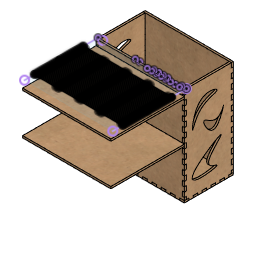
laser_skurdur_hlutur (Autodesk Fusion 360 design; units mm, degrees)
Autodesk Fusion 360 part; units mm, degrees
note: some values were not read from the file. Set by a fixed rule: which sketch regions a step uses.
sketch "botn sketch" plane through (0, 0, 0) normal (0, 0, 1) x (1, 0, 0)
  line L0 (0, 0) -> (180, 0)
  line L1 (180, 0) -> (180, 100)
  line L2 (180, 100) -> (0, 100)
  line L3 (0, 100) -> (0, 0)
  dimension "d16" = 180
  dimension "d17" = 100
  constraint horizontal L0
  constraint vertical L1
  constraint horizontal L2
  constraint vertical L3
  constraint coincident L0.start L3.end
  measures "d16" distance of L0.start L0.end
  measures "d17" distance of L0.start L2.end
extrude "Extrude1" add sketch "botn sketch" along normal blind 4 makes body 1
sketch "botn front fingur sketch" plane through (0, 0, 0) normal (0, -1, 0) x (1, 0, 0)
  line L0 (0, 0) -> (180, 0)
  line L1 (180, 0) -> (180, 4)
  line L2 (180, 4) -> (0, 4)
  line L3 (0, 4) -> (0, 0)
  line L4 (9.4737, 0) -> (18.9474, 0)
  line L5 (18.9474, 0) -> (18.9474, 4)
  line L6 (18.9474, 4) -> (9.4737, 4)
  line L7 (9.4737, 4) -> (9.4737, 0)
  dimension "d20" = 9.4737
  dimension "d21" = 9.4737
  constraint horizontal L4
  constraint vertical L5
  constraint horizontal L6
  constraint vertical L7
  constraint coincident L2 L5.end
  constraint coincident L0 L4.start
  measures "d20" distance of L5.end L6.end
  measures "d21" distance of L3 L7
extrude "Extrude2" cut sketch "botn front fingur sketch" against normal blind 4 contours L0 L2 L4 L5 L6 L7 bodies 1
pattern_linear "R-Pattern1" count 9 spacing 18.9474 along (1, 0, 0) of "Extrude2"
sketch "afturhlid sketch" plane through (0, 0, 0) normal (0, 1, 0) x (1, 0, 0)
  line L0 (0, 0) -> (180, 0)
  line L1 (180, 0) -> (180, -200)
  line L2 (180, -200) -> (0, -200)
  line L3 (0, -200) -> (0, 0)
  point P0 (180, 0)
  dimension "d28" = 200
  constraint perpendicular L0 L1
  constraint parallel L0 L2
  constraint parallel L1 L3
  constraint coincident P0 L0.end
  constraint horizontal L0
  constraint coincident L0.start L3.end
  measures "d28" distance of L0.start L2.end
extrude "Extrude3" add sketch "afturhlid sketch" along normal blind 4 separate body makes body 2
combine "Combine1" operation cut target body 2 tool bodies 1 keep tools
sketch "afturhlid vinstri sketch" plane through (0, 0, 0) normal (-1, 0, 0) x (0, -1, 0)
  line L0 (-4, 4) -> (0, 4)
  line L1 (0, 4) -> (0, 200)
  line L2 (0, 200) -> (-4, 200)
  line L3 (-4, 200) -> (-4, 4)
  line L4 (0, 9.5238) -> (-4, 9.5238)
  line L5 (-4, 9.5238) -> (-4, 19.0476)
  line L6 (-4, 19.0476) -> (0, 19.0476)
  line L7 (0, 19.0476) -> (0, 9.5238)
  dimension "d31" = 9.5238
  dimension "d32" = 9.5238
  constraint horizontal L4
  constraint vertical L5
  constraint horizontal L6
  constraint vertical L7
  constraint coincident L3 L5.end
  constraint coincident L1 L4.start
  measures "d31" distance of L4.start L6.end
  measures "d32" distance of origin L4
extrude "Extrude4" cut sketch "afturhlid vinstri sketch" against normal blind 4 contours L1 L3 L4 L5 L6 L7 bodies 2
pattern_linear "R-Pattern2" count 10 spacing 19.0476 along (0, 0, 1) of "Extrude4"
extrude "Extrude5" add 1 faces at (99.2281, 4, 106.0952) along direction (0, -1, 0) blind 4 from surface at -96 separate body on bodies 2 makes body 3
combine "Combine2" operation cut target body 1 tool bodies 3 keep tools
sketch "hlid sketch" plane through (0, 0, 0) normal (1, 0, 0) x (0, 1, 0)
  line L0 (0, 0) -> (100, 0)
  line L1 (100, 0) -> (100, 200)
  line L2 (100, 200) -> (0, 200)
  line L3 (0, 200) -> (0, 0)
  dimension "d42" = 100
  dimension "d43" = 200
  constraint horizontal L0
  constraint vertical L1
  constraint horizontal L2
  constraint vertical L3
  constraint coincident L0.start L3.end
  measures "d42" distance of L0.start L0.end
  measures "d43" distance of L0.start L2.end
extrude "Extrude6" add sketch "hlid sketch" along normal blind 4 separate body makes body 4
sketch "hlid_botn fingur sketch" plane through (0, 0, 0) normal (-1, 0, 0) x (0, -1, 0)
  line L0 (-100, 0) -> (0, 0)
  line L1 (0, 0) -> (0, 4)
  line L2 (0, 4) -> (-100, 4)
  line L3 (-100, 4) -> (-100, 0)
  line L4 (-9.0909, 0) -> (-18.1818, 0)
  line L5 (-18.1818, 0) -> (-18.1818, 4)
  line L6 (-18.1818, 4) -> (-9.0909, 4)
  line L7 (-9.0909, 4) -> (-9.0909, 0)
  dimension "d46" = 9.0909
  dimension "d47" = 9.0909
  constraint horizontal L4
  constraint vertical L5
  constraint horizontal L6
  constraint vertical L7
  constraint coincident L2 L5.end
  constraint coincident L0 L4.start
  measures "d46" distance of L4.start L4.end
  measures "d47" distance of L0.end L7
extrude "Extrude7" cut sketch "hlid_botn fingur sketch" against normal blind 4 contours L0 L2 L4 L5 L6 L7 bodies 1
pattern_linear "R-Pattern3" count 5 spacing 18.1818 along (0, 1, 0) of "Extrude7"
combine "Combine3" operation cut target body 4 tool bodies 3 2 1 keep tools
extrude "Extrude8" add 1 faces at (4, 51.5152, 33.0794) along direction (-1, 0, 0) blind 4 from surface at -176 separate body on bodies 4 makes body 5
combine "Combine4" operation cut target body 2 tool bodies 5 keep tools
combine "Combine5" operation cut target body 1 tool bodies 5 keep tools
combine "Combine6" operation cut target body 3 tool bodies 5 keep tools
sketch "living hinge fyrsta sketch" plane through (0, 4, 0) normal (0, 1, 0) x (-1, 0, 0)
  line L0 (-176, 190.4762) -> (-176, 180.9524)
  line L1 (-176, 47.619) -> (-180, 47.619)
  line L2 (-180, 180.9524) -> (-180, 171.4286)
  line L3 (-180, 38.0952) -> (-176, 38.0952)
  line L4 (-176, 38.0952) -> (-176, 28.5714)
  line L5 (-176, 28.5714) -> (-180, 28.5714)
  line L6 (-180, 28.5714) -> (-180, 19.0476)
  line L7 (-180, 19.0476) -> (-176, 19.0476)
  line L8 (-176, 19.0476) -> (-176, 9.5238)
  line L9 (-176, 9.5238) -> (-180, 9.5238)
  line L10 (-180, 9.5238) -> (-180, 4)
  line L11 (-180, 4) -> (-170.5263, 4)
  line L12 (-94.7368, 4) -> (-94.7368, 0)
  line L13 (-170.5263, 0) -> (-161.0526, 0)
  line L14 (-85.2632, 0) -> (-85.2632, 4)
  line L15 (-85.2632, 4) -> (-75.7895, 4)
  line L16 (-75.7895, 4) -> (-75.7895, 0)
  line L17 (-75.7895, 0) -> (-66.3158, 0)
  line L18 (-66.3158, 0) -> (-66.3158, 4)
  line L19 (-66.3158, 4) -> (-56.8421, 4)
  line L20 (-56.8421, 4) -> (-56.8421, 0)
  line L21 (-56.8421, 0) -> (-47.3684, 0)
  line L22 (-47.3684, 0) -> (-47.3684, 4)
  line L23 (-47.3684, 4) -> (-37.8947, 4)
  line L24 (-37.8947, 4) -> (-37.8947, 0)
  line L25 (-37.8947, 0) -> (-28.4211, 0)
  line L26 (-28.4211, 0) -> (-28.4211, 4)
  line L27 (-28.4211, 4) -> (-18.9474, 4)
  line L28 (-18.9474, 4) -> (-18.9474, 0)
  line L29 (-18.9474, 0) -> (-9.4737, 0)
  line L30 (-9.4737, 0) -> (-9.4737, 4)
  line L31 (-9.4737, 4) -> (0, 4)
  line L32 (0, 4) -> (0, 9.5238)
  line L33 (0, 9.5238) -> (-4, 9.5238)
  line L34 (-4, 9.5238) -> (-4, 19.0476)
  line L35 (-4, 19.0476) -> (0, 19.0476)
  line L36 (0, 19.0476) -> (0, 28.5714)
  line L37 (0, 28.5714) -> (-4, 28.5714)
  line L38 (-4, 28.5714) -> (-4, 38.0952)
  line L39 (-4, 38.0952) -> (0, 38.0952)
  line L40 (0, 38.0952) -> (0, 47.619)
  line L41 (0, 47.619) -> (-4, 47.619)
  line L42 (-4, 47.619) -> (-4, 57.1429)
  line L43 (-4, 57.1429) -> (0, 57.1429)
  line L44 (0, 57.1429) -> (0, 66.6667)
  line L45 (0, 200) -> (-180, 200)
  line L46 (-180, 200) -> (-180, 190.4762)
  line L47 (-180, 57.1429) -> (-176, 57.1429)
  line L48 (0, 200) -> (-180, 200)
  line L49 (-180, 200) -> (-180, 196)
  line L50 (-180, 196) -> (0, 196)
  line L51 (0, 196) -> (0, 200)
  line L52 (-176, 85.7143) -> (-180, 85.7143)
  line L53 (-180, 76.1905) -> (-176, 76.1905)
  line L54 (-176, 76.1905) -> (-176, 66.6667)
  line L55 (-176, 66.6667) -> (-180, 66.6667)
  line L56 (-180, 66.6667) -> (-180, 57.1429)
  line L57 (0, 66.6667) -> (-4, 66.6667)
  line L58 (-4, 66.6667) -> (-4, 76.1905)
  line L59 (-4, 76.1905) -> (0, 76.1905)
  line L60 (0, 76.1905) -> (0, 85.7143)
  line L61 (0, 85.7143) -> (-4, 85.7143)
  line L62 (-4, 85.7143) -> (-4, 95.2381)
  line L63 (-4, 95.2381) -> (0, 95.2381)
  line L64 (0, 95.2381) -> (0, 104.7619)
  line L65 (-180, 95.2381) -> (-176, 95.2381)
  line L66 (-176, 180.9524) -> (-180, 180.9524)
  line L67 (-180, 171.4286) -> (-176, 171.4286)
  line L68 (-176, 171.4286) -> (-176, 161.9048)
  line L69 (-176, 161.9048) -> (-180, 161.9048)
  line L70 (-180, 161.9048) -> (-180, 152.381)
  line L71 (-180, 152.381) -> (-176, 152.381)
  line L72 (-176, 152.381) -> (-176, 142.8571)
  line L73 (-176, 142.8571) -> (-180, 142.8571)
  line L74 (-180, 142.8571) -> (-180, 133.3333)
  line L75 (-180, 133.3333) -> (-176, 133.3333)
  line L76 (-176, 133.3333) -> (-176, 123.8095)
  line L77 (-176, 123.8095) -> (-180, 123.8095)
  line L78 (-180, 123.8095) -> (-180, 114.2857)
  line L79 (-180, 114.2857) -> (-176, 114.2857)
  line L80 (-176, 114.2857) -> (-176, 104.7619)
  line L81 (-176, 104.7619) -> (-180, 104.7619)
  line L82 (-180, 104.7619) -> (-180, 95.2381)
  line L83 (-176, 95.2381) -> (-176, 85.7143)
  line L84 (-180, 85.7143) -> (-180, 76.1905)
  line L85 (0, 104.7619) -> (-4, 104.7619)
  line L86 (-4, 104.7619) -> (-4, 114.2857)
  line L87 (-4, 114.2857) -> (0, 114.2857)
  line L88 (0, 114.2857) -> (0, 123.8095)
  line L89 (0, 123.8095) -> (-4, 123.8095)
  line L90 (-4, 123.8095) -> (-4, 133.3333)
  line L91 (-4, 133.3333) -> (0, 133.3333)
  line L92 (0, 133.3333) -> (0, 142.8571)
  line L93 (0, 142.8571) -> (-4, 142.8571)
  line L94 (-4, 142.8571) -> (-4, 152.381)
  line L95 (-4, 152.381) -> (0, 152.381)
  line L96 (0, 152.381) -> (0, 161.9048)
  line L97 (0, 161.9048) -> (-4, 161.9048)
  line L98 (-4, 161.9048) -> (-4, 171.4286)
  line L99 (-4, 171.4286) -> (0, 171.4286)
  line L100 (0, 171.4286) -> (0, 180.9524)
  line L101 (0, 180.9524) -> (-4, 180.9524)
  line L102 (-4, 180.9524) -> (-4, 190.4762)
  line L103 (-4, 190.4762) -> (0, 190.4762)
  line L104 (0, 190.4762) -> (0, 200)
  line L105 (-180, 190.4762) -> (-176, 190.4762)
  line L106 (-176, 57.1429) -> (-176, 47.619)
  line L107 (-180, 47.619) -> (-180, 38.0952)
  line L108 (-170.5263, 4) -> (-170.5263, 0)
  line L109 (-161.0526, 0) -> (-161.0526, 4)
  line L110 (-161.0526, 4) -> (-151.5789, 4)
  line L111 (-151.5789, 4) -> (-151.5789, 0)
  line L112 (-151.5789, 0) -> (-142.1053, 0)
  line L113 (-142.1053, 0) -> (-142.1053, 4)
  line L114 (-142.1053, 4) -> (-132.6316, 4)
  line L115 (-132.6316, 4) -> (-132.6316, 0)
  line L116 (-132.6316, 0) -> (-123.1579, 0)
  line L117 (-123.1579, 0) -> (-123.1579, 4)
  line L118 (-123.1579, 4) -> (-113.6842, 4)
  line L119 (-113.6842, 4) -> (-113.6842, 0)
  line L120 (-113.6842, 0) -> (-104.2105, 0)
  line L121 (-104.2105, 0) -> (-104.2105, 4)
  line L122 (-104.2105, 4) -> (-94.7368, 4)
  line L123 (-94.7368, 0) -> (-85.2632, 0)
  point P0 (0, 200)
  dimension "d57" = 180
  dimension "d58" = 4
  constraint horizontal L48
  constraint vertical L49
  constraint horizontal L50
  constraint vertical L51
  constraint coincident P0 L45.start
  measures "d57" distance of P0 L45.end
  measures "d58" distance of P0 L50.end
extrude "Extrude9" add sketch "living hinge fyrsta sketch" against normal blind 150 separate body contours L45 L46 L48 L49 L50 L51 L104 makes body 6
sketch "living hinge annad sketch" plane through (0, 4, 0) normal (0, 1, 0) x (-1, 0, 0)
  line L0 (0, 196) -> (0, 200)
  line L1 (0, 200) -> (-180, 200)
  line L2 (-180, 200) -> (-180, 196)
  line L3 (-180, 196) -> (0, 196)
  line L4 (-9.4737, 200) -> (-18.9474, 200)
  line L5 (-18.9474, 200) -> (-18.9474, 196)
  line L6 (-18.9474, 196) -> (-9.4737, 196)
  line L7 (-9.4737, 196) -> (-9.4737, 200)
  dimension "d62" = 9.4737
  dimension "d63" = 9.4737
  constraint horizontal L4
  constraint vertical L5
  constraint horizontal L6
  constraint vertical L7
  constraint coincident L3 L5.end
  constraint coincident L1 L4.start
  measures "d62" distance of L4.start L4.end
  measures "d63" distance of origin L7
extrude "Extrude10" cut sketch "living hinge annad sketch" against normal blind 4 contours L1 L3 L4 L5 L6 L7 bodies 6
pattern_linear "R-Pattern4" count 9 spacing 18.9474 along (1, 0, 0) of "Extrude10"
sketch "living hinge adal sketch" plane through (0, 0, 200) normal (0, 0, 1) x (-1, 0, 0)
  line L0 (-85.2632, 0) -> (-85.2632, -4)
  line L1 (-161.0526, -4) -> (-151.5789, -4)
  line L2 (-75.7895, -4) -> (-75.7895, 0)
  line L3 (-75.7895, 0) -> (-66.3158, 0)
  line L4 (-66.3158, 0) -> (-66.3158, -4)
  line L5 (-66.3158, -4) -> (-56.8421, -4)
  line L6 (-56.8421, -4) -> (-56.8421, 0)
  line L7 (-56.8421, 0) -> (-47.3684, 0)
  line L8 (-47.3684, 0) -> (-47.3684, -4)
  line L9 (-47.3684, -4) -> (-37.8947, -4)
  line L10 (-37.8947, -4) -> (-37.8947, 0)
  line L11 (-37.8947, 0) -> (-28.4211, 0)
  line L12 (-28.4211, 0) -> (-28.4211, -4)
  line L13 (-28.4211, -4) -> (-18.9474, -4)
  line L14 (-18.9474, -4) -> (-18.9474, 0)
  line L15 (-18.9474, 0) -> (-9.4737, 0)
  line L16 (-9.4737, 0) -> (-9.4737, -4)
  line L17 (-9.4737, -4) -> (0, -4)
  line L18 (0, -4) -> (0, 146) construction
  line L19 (0, 146) -> (-180, 146)
  line L20 (-180, 146) -> (-180, -4)
  line L21 (-104.2105, -4) -> (-94.7368, -4)
  line L22 (-94.7368, -4) -> (-94.7368, 0)
  line L23 (-94.7368, 0) -> (-85.2632, 0)
  line L24 (0, 26) -> (-180, 26) construction
  line L25 (0, 126) -> (-180, 126) construction
  line L26 (0, 76) -> (-180, 76) construction
  line L27 (0, -4) -> (-9.4737, -4) construction
  line L28 (-180, -4) -> (-180, 146)
  line L29 (0, -4) -> (0, 146)
  line L30 (0.5, 26) -> (-43.5, 26)
  line L31 (-49.5, 26) -> (-130.5, 26)
  line L32 (-6, 28) -> (-87, 28)
  line L33 (-93, 28) -> (-174, 28)
  line L34 (-136.5, 26) -> (-180.5, 26)
  line L35 (-90, 76) -> (-90, 26) construction
  line L36 (-46.5, 28) -> (-43.5, 26) construction
  line L37 (-46.5, 28) -> (-49.5, 26) construction
  line L38 (0.5, 126) -> (-43.5, 126)
  line L39 (-49.5, 126) -> (-130.5, 126)
  line L40 (-136.5, 126) -> (-180.5, 126)
  line L41 (0.5, 30) -> (-43.5, 30)
  line L42 (-6, 32) -> (-87, 32)
  line L43 (-49.5, 30) -> (-130.5, 30)
  line L44 (-93, 32) -> (-174, 32)
  line L45 (-136.5, 30) -> (-180.5, 30)
  line L46 (0.5, 34) -> (-43.5, 34)
  line L47 (-6, 36) -> (-87, 36)
  line L48 (-49.5, 34) -> (-130.5, 34)
  line L49 (-93, 36) -> (-174, 36)
  line L50 (-136.5, 34) -> (-180.5, 34)
  line L51 (0.5, 38) -> (-43.5, 38)
  line L52 (-6, 40) -> (-87, 40)
  line L53 (-49.5, 38) -> (-130.5, 38)
  line L54 (-93, 40) -> (-174, 40)
  line L55 (-136.5, 38) -> (-180.5, 38)
  line L56 (0.5, 42) -> (-43.5, 42)
  line L57 (-6, 44) -> (-87, 44)
  line L58 (-49.5, 42) -> (-130.5, 42)
  line L59 (-93, 44) -> (-174, 44)
  line L60 (-136.5, 42) -> (-180.5, 42)
  line L61 (0.5, 46) -> (-43.5, 46)
  line L62 (-6, 48) -> (-87, 48)
  line L63 (-49.5, 46) -> (-130.5, 46)
  line L64 (-93, 48) -> (-174, 48)
  line L65 (-136.5, 46) -> (-180.5, 46)
  line L66 (0.5, 50) -> (-43.5, 50)
  line L67 (-6, 52) -> (-87, 52)
  line L68 (-49.5, 50) -> (-130.5, 50)
  line L69 (-93, 52) -> (-174, 52)
  line L70 (-136.5, 50) -> (-180.5, 50)
  line L71 (0.5, 54) -> (-43.5, 54)
  line L72 (-6, 56) -> (-87, 56)
  line L73 (-49.5, 54) -> (-130.5, 54)
  line L74 (-93, 56) -> (-174, 56)
  line L75 (-136.5, 54) -> (-180.5, 54)
  line L76 (0.5, 58) -> (-43.5, 58)
  line L77 (-6, 60) -> (-87, 60)
  line L78 (-49.5, 58) -> (-130.5, 58)
  line L79 (-93, 60) -> (-174, 60)
  line L80 (-136.5, 58) -> (-180.5, 58)
  line L81 (0.5, 62) -> (-43.5, 62)
  line L82 (-6, 64) -> (-87, 64)
  line L83 (-49.5, 62) -> (-130.5, 62)
  line L84 (-93, 64) -> (-174, 64)
  line L85 (-136.5, 62) -> (-180.5, 62)
  line L86 (0.5, 66) -> (-43.5, 66)
  line L87 (-6, 68) -> (-87, 68)
  line L88 (-49.5, 66) -> (-130.5, 66)
  line L89 (-93, 68) -> (-174, 68)
  line L90 (-136.5, 66) -> (-180.5, 66)
  line L91 (0.5, 70) -> (-43.5, 70)
  line L92 (-6, 72) -> (-87, 72)
  line L93 (-49.5, 70) -> (-130.5, 70)
  line L94 (-93, 72) -> (-174, 72)
  line L95 (-136.5, 70) -> (-180.5, 70)
  line L96 (0.5, 74) -> (-43.5, 74)
  line L97 (-6, 76) -> (-87, 76)
  line L98 (-49.5, 74) -> (-130.5, 74)
  line L99 (-93, 76) -> (-174, 76)
  line L100 (-136.5, 74) -> (-180.5, 74)
  line L101 (0.5, 78) -> (-43.5, 78)
  line L102 (-6, 80) -> (-87, 80)
  line L103 (-49.5, 78) -> (-130.5, 78)
  line L104 (-93, 80) -> (-174, 80)
  line L105 (-136.5, 78) -> (-180.5, 78)
  line L106 (0.5, 82) -> (-43.5, 82)
  line L107 (-6, 84) -> (-87, 84)
  line L108 (-49.5, 82) -> (-130.5, 82)
  line L109 (-93, 84) -> (-174, 84)
  line L110 (-136.5, 82) -> (-180.5, 82)
  line L111 (0.5, 86) -> (-43.5, 86)
  line L112 (-6, 88) -> (-87, 88)
  line L113 (-49.5, 86) -> (-130.5, 86)
  line L114 (-93, 88) -> (-174, 88)
  line L115 (-136.5, 86) -> (-180.5, 86)
  line L116 (0.5, 90) -> (-43.5, 90)
  line L117 (-6, 92) -> (-87, 92)
  line L118 (-49.5, 90) -> (-130.5, 90)
  line L119 (-93, 92) -> (-174, 92)
  line L120 (-136.5, 90) -> (-180.5, 90)
  line L121 (0.5, 94) -> (-43.5, 94)
  line L122 (-6, 96) -> (-87, 96)
  line L123 (-49.5, 94) -> (-130.5, 94)
  line L124 (-93, 96) -> (-174, 96)
  line L125 (-136.5, 94) -> (-180.5, 94)
  line L126 (0.5, 98) -> (-43.5, 98)
  line L127 (-6, 100) -> (-87, 100)
  line L128 (-49.5, 98) -> (-130.5, 98)
  line L129 (-93, 100) -> (-174, 100)
  line L130 (-136.5, 98) -> (-180.5, 98)
  line L131 (0.5, 102) -> (-43.5, 102)
  line L132 (-6, 104) -> (-87, 104)
  line L133 (-49.5, 102) -> (-130.5, 102)
  line L134 (-93, 104) -> (-174, 104)
  line L135 (-136.5, 102) -> (-180.5, 102)
  line L136 (0.5, 106) -> (-43.5, 106)
  line L137 (-6, 108) -> (-87, 108)
  line L138 (-49.5, 106) -> (-130.5, 106)
  line L139 (-93, 108) -> (-174, 108)
  line L140 (-136.5, 106) -> (-180.5, 106)
  line L141 (0.5, 110) -> (-43.5, 110)
  line L142 (-6, 112) -> (-87, 112)
  line L143 (-49.5, 110) -> (-130.5, 110)
  line L144 (-93, 112) -> (-174, 112)
  line L145 (-136.5, 110) -> (-180.5, 110)
  line L146 (0.5, 114) -> (-43.5, 114)
  line L147 (-6, 116) -> (-87, 116)
  line L148 (-49.5, 114) -> (-130.5, 114)
  line L149 (-93, 116) -> (-174, 116)
  line L150 (-136.5, 114) -> (-180.5, 114)
  line L151 (0.5, 118) -> (-43.5, 118)
  line L152 (-6, 120) -> (-87, 120)
  line L153 (-49.5, 118) -> (-130.5, 118)
  line L154 (-93, 120) -> (-174, 120)
  line L155 (-136.5, 118) -> (-180.5, 118)
  line L156 (0.5, 122) -> (-43.5, 122)
  line L157 (-6, 124) -> (-87, 124)
  line L158 (-49.5, 122) -> (-130.5, 122)
  line L159 (-93, 124) -> (-174, 124)
  line L160 (-136.5, 122) -> (-180.5, 122)
  line L161 (-161.0526, 0) -> (-161.0526, -4)
  line L162 (-151.5789, -4) -> (-151.5789, 0)
  line L163 (-151.5789, 0) -> (-142.1053, 0)
  line L164 (-142.1053, 0) -> (-142.1053, -4)
  line L165 (-142.1053, -4) -> (-132.6316, -4)
  line L166 (-132.6316, -4) -> (-132.6316, 0)
  line L167 (-132.6316, 0) -> (-123.1579, 0)
  line L168 (-123.1579, 0) -> (-123.1579, -4)
  line L169 (-123.1579, -4) -> (-113.6842, -4)
  line L170 (-113.6842, -4) -> (-113.6842, 0)
  line L171 (-113.6842, 0) -> (-104.2105, 0)
  line L172 (-104.2105, 0) -> (-104.2105, -4)
  line L173 (-85.2632, -4) -> (-75.7895, -4)
  line L174 (-180, -4) -> (-170.5263, -4)
  line L175 (-170.5263, -4) -> (-170.5263, 0)
  line L176 (-170.5263, 0) -> (-161.0526, 0)
  dimension "d72" = 30
  dimension "d73" = 100
  dimension "d76" = 6
  dimension "d77" = 6
  dimension "d78" = 6
  dimension "d79" = 0.5
  dimension "d80" = 0.5
  dimension "d81" = 6
  dimension "d82" = 6
  dimension "d85" = 2
  dimension "d88" = 0
  dimension "d89" = 4
  constraint parallel L24 L25
  constraint parallel L25 L26
  constraint vertical L24.start L26.start
  constraint vertical L25.start L26.start
  constraint parallel L24 L27
  constraint symmetric L24 L25 L26
  constraint vertical L24.end L26.end
  constraint vertical L25.end L26.end
  constraint coincident L20 L24.end
  constraint coincident L18 L26.start
  constraint collinear L24 L30
  constraint collinear L24 L31
  constraint collinear L24 L34
  constraint midpoint L26 L35.start
  constraint perpendicular L31 L35
  constraint midpoint L31 L35.end
  constraint coincident L24 L31.start
  constraint horizontal L32
  constraint collinear L32 L33
  constraint symmetric L32.end L33.start L35
  constraint coincident L24 L30.end
  constraint midpoint L32 L36.start
  constraint equal L36 L37
  constraint symmetric L26 L30.start L38.start
  constraint symmetric L26 L30.end L38.end
  constraint symmetric L26 L31.start L39.start
  constraint symmetric L26 L31.end L39.end
  constraint symmetric L26 L34.start L40.start
  constraint symmetric L26 L34.end L40.end
  measures "d72" distance of L24 L27
  measures "d73" distance of L24 L25
  measures "d76" distance of L30.end L31.start
  measures "d77" distance of L31.end L34.start
  measures "d78" distance of L32.end L33.start
  measures "d79" distance of L24.start L30.start
  measures "d80" distance of L20 L34.end
  measures "d81" horizontal distance of L24.start L32.start
  measures "d82" horizontal distance of L24.end L33.end
  measures "d85" distance of L30 L32
sketch "list2" plane through (0, 0, 0) normal (-1, 0, 0) x (0, -1, 0)
  line L0 (-96, 4) -> (-90.9091, 4)
  line L1 (-54.5455, 4) -> (-54.5455, 0)
  line L2 (-90.9091, 0) -> (-81.8182, 0)
  line L3 (-45.4545, 0) -> (-45.4545, 4)
  line L4 (-45.4545, 4) -> (-36.3636, 4)
  line L5 (-36.3636, 4) -> (-36.3636, 0)
  line L6 (-36.3636, 0) -> (-27.2727, 0)
  line L7 (-27.2727, 0) -> (-27.2727, 4)
  line L8 (-27.2727, 4) -> (-18.1818, 4)
  line L9 (-18.1818, 4) -> (-18.1818, 0)
  line L10 (-18.1818, 0) -> (-9.0909, 0)
  line L11 (-9.0909, 0) -> (-9.0909, 4)
  line L12 (-9.0909, 4) -> (-4, 4)
  line L13 (-4, 4) -> (-4, 9.5238)
  line L14 (-4, 9.5238) -> (0, 9.5238)
  line L15 (0, 9.5238) -> (0, 19.0476)
  line L16 (0, 19.0476) -> (-4, 19.0476)
  line L17 (-4, 19.0476) -> (-4, 28.5714)
  line L18 (-4, 28.5714) -> (0, 28.5714)
  line L19 (0, 28.5714) -> (0, 38.0952)
  line L20 (0, 38.0952) -> (-4, 38.0952)
  line L21 (-4, 38.0952) -> (-4, 47.619)
  line L22 (-4, 47.619) -> (0, 47.619)
  line L23 (0, 47.619) -> (0, 57.1429)
  line L24 (0, 57.1429) -> (-4, 57.1429)
  line L25 (-4, 57.1429) -> (-4, 66.6667)
  line L26 (-4, 66.6667) -> (0, 66.6667)
  line L27 (0, 66.6667) -> (0, 76.1905)
  line L28 (0, 76.1905) -> (-4, 76.1905)
  line L29 (-4, 76.1905) -> (-4, 85.7143)
  line L30 (-4, 85.7143) -> (0, 85.7143)
  line L31 (0, 85.7143) -> (0, 95.2381)
  line L32 (0, 95.2381) -> (-4, 95.2381)
  line L33 (-4, 95.2381) -> (-4, 104.7619)
  line L34 (-4, 200) -> (-96, 200)
  line L35 (-96, 200) -> (-96, 190.4762)
  line L36 (-96, 95.2381) -> (-100, 95.2381)
  line L37 (-100, 190.4762) -> (-100, 180.9524)
  line L38 (-100, 85.7143) -> (-96, 85.7143)
  line L39 (-96, 85.7143) -> (-96, 76.1905)
  line L40 (-96, 76.1905) -> (-100, 76.1905)
  line L41 (-100, 76.1905) -> (-100, 66.6667)
  line L42 (-100, 66.6667) -> (-96, 66.6667)
  line L43 (-96, 66.6667) -> (-96, 57.1429)
  line L44 (-96, 57.1429) -> (-100, 57.1429)
  line L45 (-100, 57.1429) -> (-100, 47.619)
  line L46 (-100, 47.619) -> (-96, 47.619)
  line L47 (-96, 47.619) -> (-96, 38.0952)
  line L48 (-96, 38.0952) -> (-100, 38.0952)
  line L49 (-100, 38.0952) -> (-100, 28.5714)
  line L50 (-100, 28.5714) -> (-96, 28.5714)
  line L51 (-96, 28.5714) -> (-96, 19.0476)
  line L52 (-96, 19.0476) -> (-100, 19.0476)
  line L53 (-100, 19.0476) -> (-100, 9.5238)
  line L54 (-100, 9.5238) -> (-96, 9.5238)
  line L55 (-96, 9.5238) -> (-96, 4)
  spline S0 degree 5 poles (-66.6667, 166.6667) (-66.5889, 167.1344) (-66.0038, 168.1021) (-63.8431, 169.6256) (-58.6604, 171.4949) (-49.7639, 172.2688) (-40.1691, 170.1888) (-31.4922, 164.4289) (-24.7306, 155.2647) (-20.13, 144.139) (-17.498, 133.0535) (-16.3874, 124.1611) (-16.3352, 119.2562) (-17.0489, 119.3622) (-18.6835, 124.1124) (-21.7033, 132.0296) (-26.5802, 141.1563) (-33.5348, 149.5719) (-42.2768, 155.9219) (-51.6775, 160.0332) (-60.1178, 162.5501) (-64.7643, 164.0616) (-66.4702, 165.2955) (-66.7444, 166.1989) (-66.6667, 166.6667) knots 0 0 0 0 0 0 0.05 0.1 0.15 0.2 0.25 0.3 0.35 0.4 0.45 0.5 0.55 0.6 0.65 0.7 0.75 0.8 0.85 0.9 0.95 1 1 1 1 1 1
  spline S1 degree 5 poles (-66.6667, 116.6667) (-65.433, 116.312) (-62.8587, 115.9393) (-58.7337, 116.4236) (-53.0189, 118.8815) (-46.5036, 123.0494) (-41.6048, 125.9738) (-39.1168, 125.6797) (-39.4198, 121.4268) (-42.3138, 114.3516) (-47.223, 106.6086) (-53.3505, 100.7017) (-59.847, 98.7458) (-65.9666, 101.7694) (-71.2362, 108.9381) (-75.392, 118.2123) (-78.3126, 127.0258) (-79.9552, 132.9669) (-80.2984, 134.4017) (-79.271, 131.2681) (-76.7306, 125.4066) (-73.4219, 120.611) (-70.2605, 118.067) (-67.9003, 117.0213) (-66.6667, 116.6667) knots 0 0 0 0 0 0 0.05 0.1 0.15 0.2 0.25 0.3 0.35 0.4 0.45 0.5 0.55 0.6 0.65 0.7 0.75 0.8 0.85 0.9 0.95 1 1 1 1 1 1
  spline S2 degree 5 poles (-75, 83.3333) (-74.8425, 83.6599) (-73.8259, 83.8067) (-70.1176, 82.4615) (-61.0932, 77.6417) (-45.7669, 67.8616) (-30.2354, 56.2191) (-18.5209, 44.8127) (-13.851, 35.5225) (-17.844, 29.65) (-29.2407, 27.3859) (-44.27, 27.9032) (-58.2715, 29.9345) (-67.0147, 32.226) (-67.9671, 33.9772) (-62.0327, 35.4385) (-53.7414, 37.9657) (-48.2936, 42.9765) (-49.2179, 51.1133) (-55.9733, 61.3923) (-65.5569, 71.891) (-72.1656, 78.6367) (-74.7711, 81.8475) (-75.1575, 83.0068) (-75, 83.3333) knots 0 0 0 0 0 0 0.05 0.1 0.15 0.2 0.25 0.3 0.35 0.4 0.45 0.5 0.55 0.6 0.65 0.7 0.75 0.8 0.85 0.9 0.95 1 1 1 1 1 1
  line L56 (-45.4545, 0) -> (-36.3636, 0)
  line L57 (-100, 28.5714) -> (-100, 19.0476)
  line L58 (0, 9.5238) -> (0, 4)
  line L59 (-100, 66.6667) -> (-100, 57.1429)
  line L60 (0, 28.5714) -> (0, 19.0476)
  line L61 (-100, 47.619) -> (-100, 38.0952)
  line L62 (-100, 85.7143) -> (-100, 76.1905)
  line L63 (-100, 200) -> (-100, 190.4762)
  line L64 (-4, 104.7619) -> (0, 104.7619)
  line L65 (0, 104.7619) -> (0, 114.2857)
  line L66 (0, 114.2857) -> (-4, 114.2857)
  line L67 (-4, 114.2857) -> (-4, 123.8095)
  line L68 (-4, 123.8095) -> (0, 123.8095)
  line L69 (0, 123.8095) -> (0, 133.3333)
  line L70 (0, 133.3333) -> (-4, 133.3333)
  line L71 (-4, 133.3333) -> (-4, 142.8571)
  line L72 (-4, 142.8571) -> (0, 142.8571)
  line L73 (0, 142.8571) -> (0, 152.381)
  line L74 (0, 152.381) -> (-4, 152.381)
  line L75 (-4, 152.381) -> (-4, 161.9048)
  line L76 (-4, 161.9048) -> (0, 161.9048)
  line L77 (0, 161.9048) -> (0, 171.4286)
  line L78 (0, 171.4286) -> (-4, 171.4286)
  line L79 (-4, 171.4286) -> (-4, 180.9524)
  line L80 (-4, 180.9524) -> (0, 180.9524)
  line L81 (0, 180.9524) -> (0, 190.4762)
  line L82 (0, 190.4762) -> (-4, 190.4762)
  line L83 (-4, 190.4762) -> (-4, 200)
  line L84 (-96, 190.4762) -> (-100, 190.4762)
  line L85 (-100, 180.9524) -> (-96, 180.9524)
  line L86 (-96, 180.9524) -> (-96, 171.4286)
  line L87 (-96, 171.4286) -> (-100, 171.4286)
  line L88 (-100, 171.4286) -> (-100, 161.9048)
  line L89 (-100, 161.9048) -> (-96, 161.9048)
  line L90 (-96, 161.9048) -> (-96, 152.381)
  line L91 (-96, 152.381) -> (-100, 152.381)
  line L92 (-100, 152.381) -> (-100, 142.8571)
  line L93 (-100, 142.8571) -> (-96, 142.8571)
  line L94 (-96, 142.8571) -> (-96, 133.3333)
  line L95 (-96, 133.3333) -> (-100, 133.3333)
  line L96 (-100, 133.3333) -> (-100, 123.8095)
  line L97 (-100, 123.8095) -> (-96, 123.8095)
  line L98 (-96, 123.8095) -> (-96, 114.2857)
  line L99 (-96, 114.2857) -> (-100, 114.2857)
  line L100 (-100, 114.2857) -> (-100, 104.7619)
  line L101 (-100, 104.7619) -> (-96, 104.7619)
  line L102 (-96, 104.7619) -> (-96, 95.2381)
  line L103 (-90.9091, 4) -> (-90.9091, 0)
  line L104 (-81.8182, 0) -> (-81.8182, 4)
  line L105 (-81.8182, 4) -> (-72.7273, 4)
  line L106 (-72.7273, 4) -> (-72.7273, 0)
  line L107 (-72.7273, 0) -> (-63.6364, 0)
  line L108 (-63.6364, 0) -> (-63.6364, 4)
  line L109 (-63.6364, 4) -> (-54.5455, 4)
  line L110 (-54.5455, 0) -> (-45.4545, 0)
  line L111 (-100, 95.2381) -> (-100, 85.7143)
  point P0 (-35.7143, 166.6667)
  point P1 (-16.6667, 120)
  point P2 (-35, 150)
  point P3 (-40, 125)
  point P4 (-60, 100)
  point P5 (-80, 133.3333)
  point P6 (-16.6667, 33.3333)
  point P7 (-66.6667, 33.3333)
  point P8 (-50, 43.3333)
  dimension "d150" = 33.3333
  dimension "d151" = 33.3333
  dimension "d152" = 33.3333
  dimension "d153" = 33.3333
  dimension "d154" = 43.3333
  dimension "d155" = 83.3333
  dimension "d156" = 33.3333
  dimension "d157" = 16.6667
  dimension "d158" = 66.6667
  dimension "d159" = 75
  dimension "d160" = 83.3333
  dimension "d161" = 33.3333
  dimension "d162" = 40
  dimension "d163" = 50
  dimension "d164" = 25
  dimension "d165" = 20
  dimension "d166" = 100
  dimension "d167" = 40
  dimension "d168" = 35.7143
  dimension "d169" = 50
  dimension "d170" = 16.6667
  dimension "d171" = 80
  dimension "d172" = 33.3333
  dimension "d173" = 65
  measures "d150" distance of L10 P6
  measures "d151" distance of P7 L56
  measures "d152" distance of L34 P0
  measures "d153" distance of L34 S0.start
  measures "d154" distance of L6 P8
  measures "d155" distance of L6 S2.start
  measures "d156" distance of P7 L57
  measures "d157" distance of P6 L58
  measures "d158" distance of L34 P5
  measures "d159" distance of L34 P3
  measures "d160" distance of L34 S1.start
  measures "d161" distance of S1.start L59
  measures "d162" distance of L45 P4
  measures "d163" distance of P8 L60
  measures "d164" distance of S2.start L61
  measures "d165" distance of P5 L62
  measures "d166" distance of L6 P4
  measures "d167" distance of L27 P3
  measures "d168" distance of L31 P0
  measures "d169" distance of L34 P2
  measures "d170" distance of L27 P1
  measures "d171" distance of L34 P1
  measures "d172" distance of S0.start L63
  measures "d173" distance of P2 L62
extrude "Extrude14" cut sketch "list2" against normal up to surface (180 mm away) contours S0 | S1 | S2 bodies 4 5
sketch "Sketch14" plane through (0, 4, 0) normal (0, 1, 0) x (-1, 0, 0)
  line L0 (-176, 190.4762) -> (-176, 180.9524)
  line L1 (-176, 85.7143) -> (-180, 85.7143)
  line L2 (-180, 180.9524) -> (-180, 171.4286)
  line L3 (-180, 76.1905) -> (-176, 76.1905)
  line L4 (-176, 76.1905) -> (-176, 66.6667)
  line L5 (-176, 66.6667) -> (-180, 66.6667)
  line L6 (-180, 66.6667) -> (-180, 57.1429)
  line L7 (-180, 57.1429) -> (-176, 57.1429)
  line L8 (-176, 57.1429) -> (-176, 47.619)
  line L9 (-176, 47.619) -> (-180, 47.619)
  line L10 (-180, 47.619) -> (-180, 38.0952)
  line L11 (-180, 38.0952) -> (-176, 38.0952)
  line L12 (-176, 38.0952) -> (-176, 28.5714)
  line L13 (-176, 28.5714) -> (-180, 28.5714)
  line L14 (-180, 28.5714) -> (-180, 19.0476)
  line L15 (-180, 19.0476) -> (-176, 19.0476)
  line L16 (-176, 19.0476) -> (-176, 9.5238)
  line L17 (-176, 9.5238) -> (-180, 9.5238)
  line L18 (-180, 9.5238) -> (-180, 4)
  line L19 (-180, 4) -> (-170.5263, 4)
  line L20 (-94.7368, 4) -> (-94.7368, 0)
  line L21 (-170.5263, 0) -> (-161.0526, 0)
  line L22 (-85.2632, 0) -> (-85.2632, 4)
  line L23 (-85.2632, 4) -> (-75.7895, 4)
  line L24 (-75.7895, 4) -> (-75.7895, 0)
  line L25 (-75.7895, 0) -> (-66.3158, 0)
  line L26 (-66.3158, 0) -> (-66.3158, 4)
  line L27 (-66.3158, 4) -> (-56.8421, 4)
  line L28 (-56.8421, 4) -> (-56.8421, 0)
  line L29 (-56.8421, 0) -> (-47.3684, 0)
  line L30 (-47.3684, 0) -> (-47.3684, 4)
  line L31 (-47.3684, 4) -> (-37.8947, 4)
  line L32 (-37.8947, 4) -> (-37.8947, 0)
  line L33 (-37.8947, 0) -> (-28.4211, 0)
  line L34 (-28.4211, 0) -> (-28.4211, 4)
  line L35 (-28.4211, 4) -> (-18.9474, 4)
  line L36 (-18.9474, 4) -> (-18.9474, 0)
  line L37 (-18.9474, 0) -> (-9.4737, 0)
  line L38 (-9.4737, 0) -> (-9.4737, 4)
  line L39 (-9.4737, 4) -> (0, 4)
  line L40 (0, 4) -> (0, 9.5238)
  line L41 (0, 9.5238) -> (-4, 9.5238)
  line L42 (-4, 9.5238) -> (-4, 19.0476)
  line L43 (-4, 19.0476) -> (0, 19.0476)
  line L44 (0, 19.0476) -> (0, 28.5714)
  line L45 (0, 28.5714) -> (-4, 28.5714)
  line L46 (-4, 28.5714) -> (-4, 38.0952)
  line L47 (-4, 38.0952) -> (0, 38.0952)
  line L48 (0, 38.0952) -> (0, 47.619)
  line L49 (0, 47.619) -> (-4, 47.619)
  line L50 (-4, 47.619) -> (-4, 57.1429)
  line L51 (-4, 57.1429) -> (0, 57.1429)
  line L52 (0, 57.1429) -> (0, 66.6667)
  line L53 (0, 66.6667) -> (-4, 66.6667)
  line L54 (-4, 66.6667) -> (-4, 76.1905)
  line L55 (-4, 76.1905) -> (0, 76.1905)
  line L56 (0, 76.1905) -> (0, 85.7143)
  line L57 (0, 85.7143) -> (-4, 85.7143)
  line L58 (-4, 85.7143) -> (-4, 95.2381)
  line L59 (-4, 95.2381) -> (0, 95.2381)
  line L60 (0, 95.2381) -> (0, 104.7619)
  line L61 (0, 200) -> (-180, 200)
  line L62 (-180, 200) -> (-180, 190.4762)
  line L63 (-180, 95.2381) -> (-176, 95.2381)
  line L64 (-180, 186.2535) -> (0, 186.2535)
  line L65 (0, 186.2535) -> (0, 182.2535)
  line L66 (0, 182.2535) -> (-180, 182.2535)
  line L67 (-180, 182.2535) -> (-180, 186.2535)
  line L68 (-176, 180.9524) -> (-180, 180.9524)
  line L69 (-180, 171.4286) -> (-176, 171.4286)
  line L70 (-176, 171.4286) -> (-176, 161.9048)
  line L71 (-176, 161.9048) -> (-180, 161.9048)
  line L72 (-180, 161.9048) -> (-180, 152.381)
  line L73 (-180, 152.381) -> (-176, 152.381)
  line L74 (-176, 152.381) -> (-176, 142.8571)
  line L75 (-176, 142.8571) -> (-180, 142.8571)
  line L76 (-180, 142.8571) -> (-180, 133.3333)
  line L77 (-180, 133.3333) -> (-176, 133.3333)
  line L78 (-176, 133.3333) -> (-176, 123.8095)
  line L79 (-176, 123.8095) -> (-180, 123.8095)
  line L80 (-180, 123.8095) -> (-180, 114.2857)
  line L81 (-180, 114.2857) -> (-176, 114.2857)
  line L82 (-176, 114.2857) -> (-176, 104.7619)
  line L83 (-176, 104.7619) -> (-180, 104.7619)
  line L84 (-180, 104.7619) -> (-180, 95.2381)
  line L85 (0, 104.7619) -> (-4, 104.7619)
  line L86 (-4, 104.7619) -> (-4, 114.2857)
  line L87 (-4, 114.2857) -> (0, 114.2857)
  line L88 (0, 114.2857) -> (0, 123.8095)
  line L89 (0, 123.8095) -> (-4, 123.8095)
  line L90 (-4, 123.8095) -> (-4, 133.3333)
  line L91 (-4, 133.3333) -> (0, 133.3333)
  line L92 (0, 133.3333) -> (0, 142.8571)
  line L93 (0, 142.8571) -> (-4, 142.8571)
  line L94 (-4, 142.8571) -> (-4, 152.381)
  line L95 (-4, 152.381) -> (0, 152.381)
  line L96 (0, 152.381) -> (0, 161.9048)
  line L97 (0, 161.9048) -> (-4, 161.9048)
  line L98 (-4, 161.9048) -> (-4, 171.4286)
  line L99 (-4, 171.4286) -> (0, 171.4286)
  line L100 (0, 171.4286) -> (0, 180.9524)
  line L101 (0, 180.9524) -> (-4, 180.9524)
  line L102 (-4, 180.9524) -> (-4, 190.4762)
  line L103 (-4, 190.4762) -> (0, 190.4762)
  line L104 (0, 190.4762) -> (0, 200)
  line L105 (-180, 190.4762) -> (-176, 190.4762)
  line L106 (-176, 95.2381) -> (-176, 85.7143)
  line L107 (-180, 85.7143) -> (-180, 76.1905)
  line L108 (-170.5263, 4) -> (-170.5263, 0)
  line L109 (-161.0526, 0) -> (-161.0526, 4)
  line L110 (-161.0526, 4) -> (-151.5789, 4)
  line L111 (-151.5789, 4) -> (-151.5789, 0)
  line L112 (-151.5789, 0) -> (-142.1053, 0)
  line L113 (-142.1053, 0) -> (-142.1053, 4)
  line L114 (-142.1053, 4) -> (-132.6316, 4)
  line L115 (-132.6316, 4) -> (-132.6316, 0)
  line L116 (-132.6316, 0) -> (-123.1579, 0)
  line L117 (-123.1579, 0) -> (-123.1579, 4)
  line L118 (-123.1579, 4) -> (-113.6842, 4)
  line L119 (-113.6842, 4) -> (-113.6842, 0)
  line L120 (-113.6842, 0) -> (-104.2105, 0)
  line L121 (-104.2105, 0) -> (-104.2105, 4)
  line L122 (-104.2105, 4) -> (-94.7368, 4)
  line L123 (-94.7368, 0) -> (-85.2632, 0)
  dimension "d110" = 180
  dimension "d111" = 4
  constraint horizontal L64
  constraint vertical L65
  constraint horizontal L66
  constraint vertical L67
  constraint collinear L2 L67
  measures "d110" distance of L64.start L64.end
  measures "d111" distance of L64.start L66.end
sketch "Sketch17" plane through (0, 0, 0) normal (0, 1, 0) x (1, 0, 0)
  line L0 (0, -100) -> (180, -100)
  line L1 (180, -100) -> (180, -104)
  line L2 (180, -104) -> (0, -104)
  line L3 (0, -104) -> (0, -100)
  line L4 (0, -38.0952) -> (0, -28.5714)
  line L5 (0, -188) -> (180, -188)
  line L6 (180, -188) -> (180, -184)
  line L7 (180, -184) -> (0, -184)
  line L8 (0, -184) -> (0, -188)
  line L9 (0, -85.7143) -> (0, -76.1905)
  dimension "d128" = 4
  dimension "d129" = 180
  dimension "d130" = 4
  dimension "d131" = 180
  dimension "d132" = 100
  dimension "d133" = 80
  constraint horizontal L0
  constraint vertical L1
  constraint horizontal L2
  constraint vertical L3
  constraint collinear L3 L4
  constraint horizontal L5
  constraint vertical L6
  constraint horizontal L7
  constraint vertical L8
  constraint collinear L8 L9
  measures "d128" distance of L0.start L2.end
  measures "d129" distance of L1.end L2.end
  measures "d130" distance of L5.start L7.end
  measures "d131" distance of L5.start L5.end
  measures "d132" distance of origin L0
  measures "d133" distance of L2 L7
extrude "Extrude18" add sketch "Sketch17" along normal blind 4 and the other way blind 150 separate body makes body 7 at (120, -98.6667, 184) makes body 8 at (120, -47.3333, 100)
sketch "Sketch18" plane through (0, 4, 0) normal (0, 1, 0) x (-1, 0, 0)
  line L0 (0, 104) -> (-180, 104)
  line L1 (-180, 104) -> (-180, 100)
  line L2 (-180, 100) -> (0, 100)
  line L3 (0, 100) -> (0, 104)
  line L4 (-18.9474, 104) -> (-9.4737, 104)
  line L5 (-9.4737, 104) -> (-9.4737, 100)
  line L6 (-9.4737, 100) -> (-18.9474, 100)
  line L7 (-18.9474, 100) -> (-18.9474, 104)
  line L8 (0, 100) -> (-9.4737, 100)
  line L9 (-9.4737, 100) -> (-9.4737, 104)
  line L10 (-9.4737, 104) -> (0, 104)
  line L11 (0, 104) -> (0, 100)
  dimension "d138" = 9.4737
  dimension "d139" = 9.4737
  constraint horizontal L4
  constraint vertical L5
  constraint horizontal L6
  constraint vertical L7
  constraint coincident L2 L5.end
  constraint coincident L0 L4.start
  constraint horizontal L8
  constraint vertical L9
  constraint horizontal L10
  constraint vertical L11
  constraint coincident L2.end L3.start
  measures "d138" distance of L4.start L4.end
  measures "d139" distance of L3 L5
sketch "Sketch19" plane through (0, 4, 0) normal (0, 1, 0) x (-1, 0, 0)
  line L0 (0, 184) -> (0, 188)
  line L1 (0, 188) -> (-180, 188)
  line L2 (-180, 188) -> (-180, 184)
  line L3 (-180, 184) -> (0, 184)
  line L4 (-18.9474, 188) -> (-9.4737, 188)
  line L5 (-9.4737, 188) -> (-9.4737, 184)
  line L6 (-9.4737, 184) -> (-18.9474, 184)
  line L7 (-18.9474, 184) -> (-18.9474, 188)
  line L8 (-9.4737, 188) -> (0, 188)
  line L9 (0, 188) -> (0, 184)
  line L10 (0, 184) -> (-9.4737, 184)
  line L11 (-9.4737, 184) -> (-9.4737, 188)
  dimension "d140" = 9.4737
  dimension "d141" = 9.4737
  constraint horizontal L4
  constraint vertical L5
  constraint horizontal L6
  constraint vertical L7
  constraint coincident L3 L5.end
  constraint coincident L1 L4.start
  constraint horizontal L8
  constraint vertical L9
  constraint horizontal L10
  constraint vertical L11
  constraint coincident L0.start L3.end
  measures "d140" distance of L4.start L4.end
  measures "d141" distance of L0 L5
extrude "Extrude19" cut sketch "Sketch18" sketch "Sketch19" against normal blind 4 contours L0 L2 L3 L5 L8 L9 L10 L11 of sketch 2 contours L0 L1 L3 L5 L8 L9 L10 L11 bodies 7 8
pattern_linear "R-Pattern7" count 10 spacing 18.9474 along (1, 0, 0) of "Extrude19"
combine "Combine11" operation cut target body 2 tool bodies 8 7 keep tools
sketch "Sketch20" plane through (0, 100, 0) normal (0, 1, 0) x (-1, 0, 0)
  line L0 (-176, 9.5238) -> (-180, 9.5238)
  line L1 (-180, 9.5238) -> (-180, 4)
  line L2 (-180, 4) -> (-170.5263, 4)
  line L3 (-94.7368, 4) -> (-94.7368, 0)
  line L4 (-94.7368, 0) -> (-85.2632, 0)
  line L5 (-85.2632, 0) -> (-85.2632, 4)
  line L6 (-85.2632, 4) -> (-75.7895, 4)
  line L7 (-75.7895, 4) -> (-75.7895, 0)
  line L8 (-75.7895, 0) -> (-66.3158, 0)
  line L9 (-66.3158, 0) -> (-66.3158, 4)
  line L10 (-66.3158, 4) -> (-56.8421, 4)
  line L11 (-56.8421, 4) -> (-56.8421, 0)
  line L12 (-56.8421, 0) -> (-47.3684, 0)
  line L13 (-47.3684, 0) -> (-47.3684, 4)
  line L14 (-47.3684, 4) -> (-37.8947, 4)
  line L15 (-37.8947, 4) -> (-37.8947, 0)
  line L16 (-37.8947, 0) -> (-28.4211, 0)
  line L17 (-28.4211, 0) -> (-28.4211, 4)
  line L18 (-28.4211, 4) -> (-18.9474, 4)
  line L19 (-18.9474, 4) -> (-18.9474, 0)
  line L20 (-18.9474, 0) -> (-9.4737, 0)
  line L21 (-9.4737, 0) -> (-9.4737, 4)
  line L22 (-9.4737, 4) -> (0, 4)
  line L23 (0, 4) -> (0, 9.5238)
  line L24 (0, 9.5238) -> (-4, 9.5238)
  line L25 (-4, 9.5238) -> (-4, 19.0476)
  line L26 (-4, 19.0476) -> (0, 19.0476)
  line L27 (0, 19.0476) -> (0, 28.5714)
  line L28 (0, 28.5714) -> (-4, 28.5714)
  line L29 (-4, 28.5714) -> (-4, 38.0952)
  line L30 (-4, 38.0952) -> (0, 38.0952)
  line L31 (0, 38.0952) -> (0, 47.619)
  line L32 (0, 47.619) -> (-4, 47.619)
  line L33 (-4, 47.619) -> (-4, 57.1429)
  line L34 (-4, 57.1429) -> (0, 57.1429)
  line L35 (0, 57.1429) -> (0, 66.6667)
  line L36 (0, 66.6667) -> (-4, 66.6667)
  line L37 (-4, 66.6667) -> (-4, 76.1905)
  line L38 (-4, 76.1905) -> (0, 76.1905)
  line L39 (0, 76.1905) -> (0, 85.7143)
  line L40 (0, 85.7143) -> (-4, 85.7143)
  line L41 (-4, 85.7143) -> (-4, 95.2381)
  line L42 (-4, 95.2381) -> (0, 95.2381)
  line L43 (0, 190.4762) -> (0, 200)
  line L44 (0, 200) -> (-180, 200)
  line L45 (-180, 104.7619) -> (-180, 95.2381)
  line L46 (-180, 95.2381) -> (-176, 95.2381)
  line L47 (-176, 190.4762) -> (-176, 180.9524)
  line L48 (-176, 85.7143) -> (-180, 85.7143)
  line L49 (-180, 85.7143) -> (-180, 76.1905)
  line L50 (-180, 76.1905) -> (-176, 76.1905)
  line L51 (-176, 76.1905) -> (-176, 66.6667)
  line L52 (-176, 66.6667) -> (-180, 66.6667)
  line L53 (-180, 66.6667) -> (-180, 57.1429)
  line L54 (-180, 57.1429) -> (-176, 57.1429)
  line L55 (-176, 57.1429) -> (-176, 47.619)
  line L56 (-176, 47.619) -> (-180, 47.619)
  line L57 (-180, 47.619) -> (-180, 38.0952)
  line L58 (-180, 38.0952) -> (-176, 38.0952)
  line L59 (-176, 38.0952) -> (-176, 28.5714)
  line L60 (-176, 28.5714) -> (-180, 28.5714)
  line L61 (-180, 28.5714) -> (-180, 19.0476)
  line L62 (-180, 19.0476) -> (-176, 19.0476)
  line L63 (-176, 19.0476) -> (-176, 9.5238)
  line L64 (0, 95.2381) -> (0, 104.7619)
  line L65 (0, 104.7619) -> (-4, 104.7619)
  line L66 (-4, 104.7619) -> (-4, 114.2857)
  line L67 (-4, 114.2857) -> (0, 114.2857)
  line L68 (0, 114.2857) -> (0, 123.8095)
  line L69 (0, 123.8095) -> (-4, 123.8095)
  line L70 (-4, 123.8095) -> (-4, 133.3333)
  line L71 (-4, 133.3333) -> (0, 133.3333)
  line L72 (0, 133.3333) -> (0, 142.8571)
  line L73 (0, 142.8571) -> (-4, 142.8571)
  line L74 (-4, 142.8571) -> (-4, 152.381)
  line L75 (-4, 152.381) -> (0, 152.381)
  line L76 (0, 152.381) -> (0, 161.9048)
  line L77 (0, 161.9048) -> (-4, 161.9048)
  line L78 (-4, 161.9048) -> (-4, 171.4286)
  line L79 (-4, 171.4286) -> (0, 171.4286)
  line L80 (0, 171.4286) -> (0, 180.9524)
  line L81 (0, 180.9524) -> (-4, 180.9524)
  line L82 (-4, 180.9524) -> (-4, 190.4762)
  line L83 (-4, 190.4762) -> (0, 190.4762)
  line L84 (-180, 200) -> (-180, 190.4762)
  line L85 (-180, 190.4762) -> (-176, 190.4762)
  line L86 (-176, 180.9524) -> (-180, 180.9524)
  line L87 (-180, 180.9524) -> (-180, 171.4286)
  line L88 (-180, 171.4286) -> (-176, 171.4286)
  line L89 (-176, 171.4286) -> (-176, 161.9048)
  line L90 (-176, 161.9048) -> (-180, 161.9048)
  line L91 (-180, 161.9048) -> (-180, 152.381)
  line L92 (-180, 152.381) -> (-176, 152.381)
  line L93 (-176, 152.381) -> (-176, 142.8571)
  line L94 (-176, 142.8571) -> (-180, 142.8571)
  line L95 (-180, 142.8571) -> (-180, 133.3333)
  line L96 (-180, 133.3333) -> (-176, 133.3333)
  line L97 (-176, 133.3333) -> (-176, 123.8095)
  line L98 (-176, 123.8095) -> (-180, 123.8095)
  line L99 (-180, 123.8095) -> (-180, 114.2857)
  line L100 (-180, 114.2857) -> (-176, 114.2857)
  line L101 (-176, 114.2857) -> (-176, 104.7619)
  line L102 (-176, 104.7619) -> (-180, 104.7619)
  line L103 (-170.5263, 4) -> (-170.5263, 0)
  line L104 (-170.5263, 0) -> (-161.0526, 0)
  line L105 (-161.0526, 0) -> (-161.0526, 4)
  line L106 (-161.0526, 4) -> (-151.5789, 4)
  line L107 (-151.5789, 4) -> (-151.5789, 0)
  line L108 (-151.5789, 0) -> (-142.1053, 0)
  line L109 (-142.1053, 0) -> (-142.1053, 4)
  line L110 (-142.1053, 4) -> (-132.6316, 4)
  line L111 (-132.6316, 4) -> (-132.6316, 0)
  line L112 (-132.6316, 0) -> (-123.1579, 0)
  line L113 (-123.1579, 0) -> (-123.1579, 4)
  line L114 (-123.1579, 4) -> (-113.6842, 4)
  line L115 (-113.6842, 4) -> (-113.6842, 0)
  line L116 (-113.6842, 0) -> (-104.2105, 0)
  line L117 (-104.2105, 0) -> (-104.2105, 4)
  line L118 (-104.2105, 4) -> (-94.7368, 4)
  line L119 (-176, 95.2381) -> (-176, 85.7143)
hidden bodies 6
equation "hæð = 200 mm"
equation "breidd = 100 mm"
equation "lengd = 180 mm"
equation "efni = 4 mm"
equation "n_l_fingur = 9"
equation "n_b_fingur = 5"
equation "n_h_fingur = 10"
equation "l_fingur_breidd = lengd / ( ( n_l_fingur * 2 ) + 1 )"
equation "b_fingur_breidd = breidd / ( ( n_b_fingur * 2 ) + 1 )"
equation "h_fingur_breidd = hæð / ( ( n_h_fingur * 2 ) + 1 )"
equation "d16 = lengd"
equation "d17 = breidd"
equation "d18 = efni"
equation "d20 = l_fingur_breidd"
equation "d21 = l_fingur_breidd"
equation "d22 = -efni"
equation "d24 = n_l_fingur"
equation "d26 = lengd - ( 3 * l_fingur_breidd )"
equation "d28 = hæð"
equation "d29 = efni"
equation "d31 = h_fingur_breidd"
equation "d32 = h_fingur_breidd"
equation "d33 = -efni"
equation "d35 = n_h_fingur"
equation "d37 = hæð - ( h_fingur_breidd * 3 )"
equation "d40 = -efni"
equation "d42 = breidd"
equation "d43 = hæð"
equation "d44 = efni"
equation "d46 = b_fingur_breidd"
equation "d47 = b_fingur_breidd"
equation "d48 = -efni"
equation "d50 = n_b_fingur"
equation "d52 = -( breidd - ( b_fingur_breidd * 3 ) )"
equation "d55 = -efni"
equation "d57 = lengd"
equation "d58 = efni"
equation "snap_lengd = 150 mm"
equation "d60 = -snap_lengd"
equation "d62 = l_fingur_breidd"
equation "d63 = l_fingur_breidd"
equation "d64 = -efni"
equation "d66 = n_l_fingur"
equation "d68 = -( lengd - ( l_fingur_breidd * 3 ) )"
equation "pattern_heildar_hæð = 100 mm"
equation "offset_pattern = snap_lengd * 0.2"
equation "d72 = offset_pattern"
equation "d73 = pattern_heildar_hæð"
equation "lag_gap = 6 mm"
equation "kerf = 0.105 mm"
equation "d76 = lag_gap"
equation "d77 = lag_gap"
equation "d78 = lag_gap"
equation "d81 = lag_gap"
equation "d82 = lag_gap"
equation "lodrettgap = pattern_heildar_hæð / n_lodrett_gaps"
equation "n_lodrett_gaps = 50"
equation "d85 = lodrettgap"
equation "d87 = n_lodrett_gaps / 2"
equation "d89 = lodrettgap * 2"
equation "nyttbil = 80 mm"
equation "haed_fra_botn = hæð / 2"
equation "d110 = lengd"
equation "d128 = efni"
equation "d129 = lengd"
equation "d130 = efni"
equation "d131 = lengd"
equation "d132 = haed_fra_botn"
equation "d133 = nyttbil"
equation "d134 = efni"
equation "d136 = snap_lengd"
equation "d138 = l_fingur_breidd"
equation "d139 = l_fingur_breidd"
equation "d140 = l_fingur_breidd"
equation "d141 = l_fingur_breidd"
equation "d142 = -efni"
equation "d144 = n_l_fingur + 1"
equation "d146 = -( lengd - ( l_fingur_breidd ) )"
equation "list1 = hæð / 6"
equation "list2 = breidd / 3"
equation "d150 = list1"
equation "d151 = list1"
equation "d152 = list1"
equation "d153 = list1"
equation "d154 = list1 + 10 mm"
equation "d155 = list1 * 2.5"
equation "d156 = list2"
equation "d157 = list2 / 2"
equation "d158 = list1 * 2"
equation "d159 = list1 * 2.25"
equation "d160 = list1 * 2.5"
equation "d161 = breidd / 3"
equation "d162 = breidd / 2.5"
equation "d163 = breidd / 2"
equation "d164 = breidd / 4"
equation "d165 = breidd / 5"
equation "d166 = hæð / 2"
equation "d167 = breidd / 2.5"
equation "d168 = breidd / 2.8"
equation "d169 = hæð / 4"
equation "d170 = breidd / 6"
equation "d171 = hæð / 2.5"
equation "d172 = breidd / 3"
equation "d173 = breidd * 0.65"
named bodies: "botn", "afturhlid", "framhlid", "hægri hlid"
